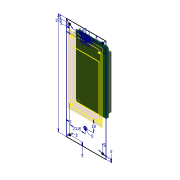
# Autodesk Inventor part: VER.2 LCD
Saved by Autodesk Inventor 2016 (Build 200138000, 138)
## iProperties
Created: 2017-12-27
Part Number: VER.2 LCD
Material: Generic
Document SubType Name: Modeling
Designer: Juny
Density: 1 g/cm^3
Appearance: Default
Author: Juny
Autodesk Inventor part; units mm, degrees
ref_plane "YZ Plane" through (0, 0, 0) normal (1, 0, 0) x (0, 1, 0)
ref_plane "XZ Plane" through (0, 0, 0) normal (0, 1, 0) x (-1, 0, 0)
ref_plane "XY Plane" through (0, 0, 0) normal (0, 0, 1) x (1, 0, 0)
sketch "Sketch1" plane through (0, 0, 0) normal (0, 1, 0) x (-1, 0, 0)
  line L0 (3.2, 0) -> (44.4, 0)
  line L1 (47.6, 3.2) -> (47.6, 91.8)
  line L2 (44.4, 95) -> (3.2, 95)
  line L3 (0, 91.8) -> (0, 3.2)
  arc A0 (47.6, 91.8) -> (44.4, 95) centre (44.4, 91.8) ccw
  arc A1 (3.2, 95) -> (0, 91.8) centre (3.2, 91.8) ccw
  arc A2 (0, 3.2) -> (3.2, 0) centre (3.2, 3.2) ccw
  arc A3 (44.4, 0) -> (47.6, 3.2) centre (44.4, 3.2) ccw
  circle A4 centre (44.4, 91.8) radius 1.6
  circle A5 centre (3.2, 91.8) radius 1.6
  circle A6 centre (44.4, 3.2) radius 1.6
  circle A7 centre (3.2, 3.2) radius 1.6
  point P0 (0, 0)
  point P1 (47.6, 95)
  point P2 (47.6, 0)
  point P3 (0, 95)
  dimension "d0" = 47.6
  dimension "d1" = 95
  dimension "d2" = 3.2
  dimension "d3" = 3.2
  dimension "d4" = 3.2
  dimension "d5" = 3.2
  dimension "d6" = 3.2
  constraints: 8 centre point, 8 end point, 8 point on circle, 8 point on line, 8 tangent, 4 coincident, 3 equal radius, 2 parallel, 1 horizontal, 1 perpendicular
  measures "d0" distance of point (47.6, 95) point (0, 95)
  measures "d1" distance of point (47.6, 0) point (47.6, 95)
  measures "d2" radius of A0
  measures "d3" diameter of A4
  measures "d4" diameter of A5
  measures "d5" diameter of A6
  measures "d6" diameter of A7
extrude "Extrusion1" add sketch "Sketch1" along normal blind 1.6
sketch "Sketch2" plane through (0, 1.6, 0) normal (0, 1, 0) x (1, 0, 0)
  circle A0 centre (-3.2, -3.2) radius 1.6 projected
  circle A1 centre (-44.4, -3.2) radius 1.6 projected
  circle A2 centre (-3.2, -91.8) radius 1.6 projected
  circle A3 centre (-44.4, -91.8) radius 1.6 projected
  line L0 (-44.4, -95) -> (-3.2, -95) projected
  arc A4 (-3.2, -95) -> (0, -91.8) centre (-3.2, -91.8) ccw projected
  line L1 (0, -91.8) -> (0, -3.2) projected
  arc A5 (0, -3.2) -> (-3.2, 0) centre (-3.2, -3.2) ccw projected
  line L2 (-3.2, 0) -> (-44.4, 0) projected
  arc A6 (-44.4, 0) -> (-47.6, -3.2) centre (-44.4, -3.2) ccw projected
  line L3 (-47.6, -3.2) -> (-47.6, -91.8) projected
  arc A7 (-47.6, -91.8) -> (-44.4, -95) centre (-44.4, -91.8) ccw projected
  line L4 (-47.6, -87.95) -> (0, -87.95)
  line L5 (0, -87.95) -> (0, -7.05)
  line L6 (0, -7.05) -> (-47.6, -7.05)
  line L7 (-47.6, -7.05) -> (-47.6, -87.95)
  point P0 (0, 0)
  dimension "d9" = 7.05
  dimension "d10" = 7.05
  constraints: 8 end point, 2 parallel, 2 point on line, 1 horizontal, 1 perpendicular
  measures "d9" distance between parallel lines of L2 L6
  measures "d10" distance between parallel lines of L0 L4
extrude "Extrusion2" add sketch "Sketch2" along normal blind 2.8 separate body contours L3 L6 L1 L4
sketch "Sketch3" plane through (0, 4.4, 0) normal (0, 1, 0) x (1, 0, 0)
  line L0 (0, -7.05) -> (-47.6, -7.05) projected
  line L1 (-47.6, -7.05) -> (-47.6, -87.95) projected
  line L2 (-47.6, -87.95) -> (0, -87.95) projected
  line L3 (0, -87.95) -> (0, -7.05) projected
  line L4 (-47.6, -3.2) -> (-47.6, -91.8) projected
  line L5 (-47.6, -85.95) -> (0, -85.95)
  point P0 (0, 0)
  dimension "d13" = 2
  constraints: 2 end point, 2 point on line, 1 perpendicular
  measures "d13" distance between parallel lines of L2 L5
extrude "Extrusion3" add sketch "Sketch3" along normal blind 1.2 separate body contours L3 L5 L1 L0
sketch "Sketch4" plane through (0, 5.6, 0) normal (0, 1, 0) x (1, 0, 0)
  line L0 (0, -7.05) -> (-47.6, -7.05) projected
  line L1 (-47.6, -7.05) -> (-47.6, -85.95) projected
  line L2 (-47.6, -85.95) -> (0, -85.95) projected
  line L3 (0, -85.95) -> (0, -7.05) projected
  line L4 (-44.4, -79.57) -> (-3.2, -79.57)
  line L5 (-3.2, -79.57) -> (-3.2, -9.97)
  line L6 (-3.2, -9.97) -> (-44.4, -9.97)
  line L7 (-44.4, -9.97) -> (-44.4, -79.57)
  line L8 (0, -7.05) -> (-47.6, -7.05) projected
  point P0 (0, 0)
  point P1 (-23.8, -7.05)
  point P2 (-23.8, -9.97)
  dimension "d16" = 2.92
  dimension "d17" = 69.6
  dimension "d18" = 41.2
  dimension "d19" = 0
  constraints: 8 end point, 2 midpoint, 2 parallel, 1 horizontal, 1 perpendicular
  measures "d16" distance between parallel lines of L0 L6
  measures "d17" distance between parallel lines of L4 L6
  measures "d18" distance between parallel lines of L5 L7
  measures "d19" horizontal distance of point (-23.8, -7.05) point (-23.8, -9.97)
extrude "Extrusion4" add sketch "Sketch4" along normal blind 0.1 separate body contours L7 L6 L5 L4
ref_plane "Work Plane1" through (0, -10, 0) normal (0, -1, 0) x (1, 0, 0)
sketch "Sketch5" plane through (0, -10, 0) normal (0, -1, 0) x (1, 0, 0)
  circle A0 centre (-3.2, 3.2) radius 1.6 projected
  circle A1 centre (-44.4, 3.2) radius 1.6 projected
  circle A2 centre (-3.2, 91.8) radius 1.6 projected
  circle A3 centre (-44.4, 91.8) radius 1.6 projected
  line L0 (-44.4, 95) -> (-3.2, 95) projected
  arc A4 (0, 91.8) -> (-3.2, 95) centre (-3.2, 91.8) ccw projected
  line L1 (0, 91.8) -> (0, 3.2) projected
  arc A5 (-3.2, 0) -> (0, 3.2) centre (-3.2, 3.2) ccw projected
  line L2 (-3.2, 0) -> (-44.4, 0) projected
  arc A6 (-47.6, 3.2) -> (-44.4, 0) centre (-44.4, 3.2) ccw projected
  line L3 (-47.6, 3.2) -> (-47.6, 91.8) projected
  arc A7 (-44.4, 95) -> (-47.6, 91.8) centre (-44.4, 91.8) ccw projected
  line L4 (-52.6, 111.7201) -> (7.4, 111.7201)
  line L5 (7.4, 111.7201) -> (7.4, -43.2799)
  line L6 (7.4, -43.2799) -> (-52.6, -43.2799)
  line L7 (-52.6, -43.2799) -> (-52.6, 111.7201)
  circle A8 centre (-47.6, 106.7201) radius 1.5
  circle A9 centre (2.4, 106.7201) radius 1.5
  circle A10 centre (-47.6, -38.2799) radius 1.5
  circle A11 centre (2.4, -38.2799) radius 1.5
  circle A12 centre (-23.8, -18) radius 2.5
  line L8 (-31.1, 105.2) -> (-16.5, 105.2)
  line L9 (-16.5, 105.2) -> (-16.5, 98)
  line L10 (-16.5, 98) -> (-31.1, 98)
  line L11 (-31.1, 98) -> (-31.1, 105.2)
  line L12 (-30.05, 104.15) -> (-17.55, 104.15)
  line L13 (-17.55, 104.15) -> (-17.55, 99.05)
  line L14 (-17.55, 99.05) -> (-30.05, 99.05)
  line L15 (-30.05, 99.05) -> (-30.05, 104.15)
  line L16 (-44.4, 95) -> (-3.2, 95) projected
  line L17 (-44.4, 79.57) -> (-3.2, 79.57) projected
  line L18 (-3.2, 79.57) -> (-3.2, 9.97) projected
  line L19 (-3.2, 9.97) -> (-44.4, 9.97) projected
  line L20 (-44.4, 9.97) -> (-44.4, 79.57) projected
  circle A13 centre (-27.3, 100.35) radius 0.46
  circle A14 centre (-24.8, 100.35) radius 0.46
  circle A15 centre (-22.8, 100.35) radius 0.46
  circle A16 centre (-20.3, 100.35) radius 0.46
  circle A17 centre (-30.45, 102.75) radius 1.15
  circle A18 centre (-17.15, 102.75) radius 1.15
  point P0 (0, 0)
  point P1 (-31.1, 101.6)
  point P2 (-30.05, 101.6)
  point P3 (-23.8, 99.05)
  point P4 (-23.8, 98)
  point P5 (-23.8, 95)
  dimension "d23" = 155
  dimension "d24" = 60
  dimension "d25" = 5
  dimension "d26" = 3
  dimension "d27" = 5
  dimension "d28" = 5
  dimension "d29" = 3
  dimension "d30" = 5
  dimension "d31" = 5
  dimension "d32" = 3
  dimension "d33" = 3
  dimension "d34" = 5
  dimension "d35" = 5
  dimension "d36" = 5
  dimension "d37" = 5
  dimension "d38" = 5
  dimension "d39" = 23.8
  dimension "d40" = 18
  dimension "d41" = 14.6
  dimension "d42" = 7.2
  dimension "d43" = 12.5
  dimension "d44" = 5.1
  dimension "d45" = 0
  dimension "d46" = 0
  dimension "d47" = 0
  dimension "d48" = 0.92
  dimension "d49" = 0.92
  dimension "d50" = 0.92
  dimension "d51" = 0.92
  dimension "d52" = 2
  dimension "d53" = 2.5
  dimension "d54" = 2.5
  dimension "d55" = 1
  dimension "d56" = 2.3
  dimension "d57" = 2.3
  dimension "d58" = 13.3
  dimension "d59" = 6.65
  dimension "d60" = 2.4
  dimension "d61" = 2.4
  dimension "d62" = 1.3
  dimension "d63" = 1.3
  dimension "d64" = 1.3
  dimension "d65" = 1.3
  dimension "d66" = 3
  constraints: 24 end point, 11 centre point, 6 parallel, 5 midpoint, 3 horizontal, 3 perpendicular
  measures "d23" distance between parallel lines of L4 L6
  measures "d24" distance between parallel lines of L5 L7
  measures "d25" distance between parallel lines of L3 L7
  measures "d26" diameter of A8
  measures "d27" distance from line of L7 A8.centre
  measures "d28" distance from line of L4 A8.centre
  measures "d29" diameter of A9
  measures "d30" distance from line of L5 A9.centre
  measures "d31" distance from line of L4 A9.centre
  measures "d32" diameter of A10
  measures "d33" diameter of A11
  measures "d34" distance from line of L5 A11.centre
  measures "d35" distance from line of L6 A11.centre
  measures "d36" distance from line of L6 A10.centre
  measures "d37" distance from line of L7 A10.centre
  measures "d38" diameter of A12
  measures "d39" distance from line of L3 A12.centre
  measures "d40" distance from line of L2 A12.centre
  measures "d41" distance of L9.end L10.end
  measures "d42" distance of L8.end L9.end
  measures "d43" distance of L13.end L14.end
  measures "d44" distance of L12.end L13.end
  measures "d45" horizontal distance of point (-23.8, 99.05) point (-23.8, 98)
  measures "d46" vertical distance of point (-31.1, 101.6) point (-30.05, 101.6)
  measures "d47" horizontal distance of point (-23.8, 98) point (-23.8, 95)
  measures "d48" diameter of A13
  measures "d49" diameter of A14
  measures "d50" diameter of A15
  measures "d51" diameter of A16
  measures "d52" distance of A14.centre A15.centre
  measures "d53" distance of A13.centre A14.centre
  measures "d54" distance of A16.centre A15.centre
  measures "d55" horizontal distance of point (-23.8, 99.05) A14.centre
  measures "d56" diameter of A17
  measures "d57" diameter of A18
  measures "d58" distance of A18.centre A17.centre
  measures "d59" horizontal distance of point (-23.8, 99.05) A17.centre
  measures "d60" vertical distance of A16.centre A18.centre
  measures "d61" vertical distance of A13.centre A17.centre
  measures "d62" vertical distance of point (-23.8, 99.05) A13.centre
  measures "d63" distance from line of L14 A14.centre
  measures "d64" distance from line of L14 A15.centre
  measures "d65" distance from line of L14 A16.centre
  measures "d66" distance between parallel lines of L0 L10
body "Solid1"
body "Solid2"
body "Solid3"
body "Solid4"
